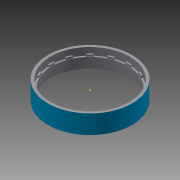
# Autodesk Inventor part: tire 2
Saved by Autodesk Inventor 2015 (Build 190159000, 159)
## iProperties
Created: 2014-10-30
Part Number: tire 2
Material: Generic
Document SubType Name: Modeling
Designer: hlorenson909
Density: 1 g/cm^3
Appearance: Default
Author: hlorenson909
Autodesk Inventor part; units mm, degrees
ref_plane "YZ Plane" through (0, 0, 0) normal (1, 0, 0) x (0, 1, 0)
ref_plane "XZ Plane" through (0, 0, 0) normal (0, 1, 0) x (-1, 0, 0)
sketch "Sketch1" plane through (0, 0, 0) normal (0, 0, 1) x (1, 0, 0)
  circle A0 centre (0, 0) radius 22.455
  circle A1 centre (0, 0) radius 21.0903
  dimension "d0" = 44.91
  constraints: 2 centre point, 1 coincident
  measures "d0" diameter of A0
extrude "Extrusion1" add sketch "Sketch1" against normal blind 10
ref_plane "Work Plane1" through (0, 0, -5) normal (0, 0, 1) x (1, 0, 0)
sketch "Sketch2" plane through (0, 0, -5) normal (0, 0, 1) x (1, 0, 0)
  circle A0 centre (0, 0) radius 21.0903 projected
  line L0 (0, 0) -> (21.0903, 0) construction
  line L1 (0, 0) -> (94, 0) construction
  arc A1 (1.418, 20.2788) -> (-1.418, 20.2788) centre (0, 0) ccw
  line L2 (1.418, 20.2788) -> (1.4712, 21.0389)
  line L3 (0, 0) -> (21.0903, 0) construction
  line L4 (-1.418, 20.2788) -> (-1.4712, 21.0389)
  line L5 (0, 0) -> (21.0903, 0) construction
  dimension "d6" = 0.762
  constraints: 12 end point, 4 horizontal, 4 point on circle, 1 centre point
  measures "d6" radial gap between concentric circles of A0 A1
extrude "Extrusion2" add sketch "Sketch2" along normal mid plane 4 contours L2 A1 L4 A0 picked at (0.1577, 20.8307)
pattern_circular "Circular Pattern1" count 16 over 360 about axis through (0, 0, 0) along (0, 0, -1) of "Extrusion2"
sketch "Sketch3" plane through (0, 0, -5) normal (0, 0, 1) x (1, 0, 0)
  point P0 (0, 0)
sketch "Sketch4" plane through (0, 0, -5) normal (0, 0, 1) x (1, 0, 0)
  circle A0 centre (0, 0) radius 21.0903 projected
  circle A1 centre (0, 0) radius 20.2448
  constraints: 1 centre point
extrude "Extrusion3" add sketch "Sketch4" along normal mid plane 2
body "Solid1"
